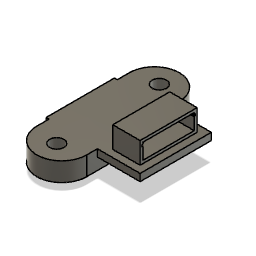
TOF_2D v1 (Autodesk Fusion 360 design; units mm, degrees)
Autodesk Fusion 360 part; units mm, degrees
note: some values were not read from the file. Set by a fixed rule: which sketch regions a step uses.
sketch "草图1" plane through (0, 0, 0) normal (0, 1, 0) x (1, 0, 0)
  line L0 (0, 0) -> (5, 0)
  line L1 (5, 0) -> (5, 9.6)
  line L2 (5, 9.6) -> (0, 9.6)
  line L3 (0, 9.6) -> (0, 0)
  circle A0 centre (2.5, 2.5) radius 2.5
  circle A1 centre (2.5, 7.1) radius 2.5
  dimension "d1" = 5
  dimension "d2" = 9.6
  dimension "d3" = 5
  dimension "d4" = 5
  constraint horizontal L0
  constraint vertical L1
  constraint horizontal L2
  constraint vertical L3
  constraint coincident L0.start L3.end
  constraint tangent L0 A0
  constraint tangent L2 A1
  constraint tangent L1 A1
  measures "d1" distance of L0.start L0.end
  measures "d2" distance of L0.start L2.end
  measures "d3" diameter of A0
  measures "d4" diameter of A1
extrude "拉伸1" add sketch "草图1" along normal blind 1 contours A0 A1 | L3 A0 A1 | L1 A0 A1 | A0 A1 | A0 A1
sketch "草图2" plane through (0, 1, 0) normal (0, 1, 0) x (-1, 0, 0)
  line L0 (1.0001, 5.2) -> (-5.9999, 5.2)
  line L1 (-5.9999, 5.2) -> (-5.9999, -14.8)
  line L2 (-5.9999, -14.8) -> (1.0001, -14.8)
  line L3 (1.0001, -14.8) -> (1.0001, 5.2)
  line L4 (8, -4.8) -> (-8, -4.8)
  line L5 (0, -7.1) -> (0, -2.5)
  line L6 (-2.4999, 15.7777) -> (-2.4999, -15.7777)
  arc A0 (0, -2.5) -> (-5, -2.4998) centre (-2.5, -2.5) ccw
  line L7 (-5.9999, 5.2) -> (1.0001, -14.8)
  line L8 (1.0001, 5.2) -> (-5.9999, -14.8)
  circle A1 centre (-2.4999, -4.8) radius 1.267
  circle A2 centre (-2.4999, -4.8) radius 1.114
  circle A3 centre (-2.4999, 1.7) radius 3.5
  circle A4 centre (-2.4999, -11.3) radius 3.5
  line L9 (1.0001, 5.2) -> (1.0001, 0)
  line L10 (1.0001, 0) -> (1.4001, 0)
  line L11 (1.4001, 0) -> (1.4001, -9.6)
  line L12 (1.4001, -9.6) -> (1.0001, -9.6)
  dimension "d11" = 7
  dimension "d12" = 20
  dimension "d13" = 7
  dimension "d14" = 7
  dimension "d15" = 5.2
  dimension "d19" = 0.4
  dimension "d20" = 9.6
  constraint horizontal L0
  constraint vertical L1
  constraint horizontal L2
  constraint vertical L3
  constraint perpendicular L1 L4
  constraint midpoint L4 L5
  constraint vertical L6
  constraint midpoint L6 A0
  constraint midpoint L8 A1.centre
  constraint coincident L6 A1.centre
  constraint coincident L4 A1.centre
  constraint concentric A1 A2
  constraint tangent L3 A3
  constraint tangent L0 A3
  constraint tangent L3 A4
  constraint tangent L2 A4
  constraint perpendicular L0 L9
  constraint perpendicular L3 L10
  constraint perpendicular L4 L11
  constraint coincident L3 L12.end
  constraint perpendicular L3 L12
  measures "d11" distance of L0.start L0.end
  measures "d12" distance of L0.start L2.end
  measures "d13" diameter of A3
  measures "d14" diameter of A4
  measures "d15" distance of L0.start L9.end
  measures "d19" distance of L9.end L10.end
  measures "d20" distance of L10.end L11.end
extrude "拉伸2" add sketch "草图2" along normal blind 2.65 contours L6 A0 L8 A3 | L6 A0 L7 A3 | A0 L8 A3 | L3 L4 L5 A0 A3 L9 | L6 A0 L8 A3 | L6 A0 L7 A3 | A0 L7 A3 | A0 L8 A3 | L4 L5 A0 L8 A1 A3 | L1 L4 L7 A1 A3 | L6 L8 A1 A3 | L6 L7 A1 A3 | A0 L7 A3 | L3 L4 L7 A1 A4 | L1 L4 L8 A1 A4 | L6 L8 A1 A2 | L6 L7 A1 A2 | L4 L8 A1 A2 | L8 A4 | L4 L7 A1 A2 | L4 L8 A1 A2 | L6 L8 A2 | L6 L7 A2 | L7 A4 | L4 L7 A1 A2 | L4 L8 A2 | L6 L8 A4 | L6 L8 A1 A4 | L4 L7 A2 | L4 L8 A2 | L6 L8 A1 A2 | L6 L7 A2 | L4 L7 A2 | L6 L8 A2 | L6 L7 A1 A4 | L6 L7 A4 | L6 L7 A1 A2
sketch "草图3" plane through (0, 3.65, 0) normal (0, 1, 0) x (-1, 0, 0)
  arc A0 (1.0001, 1.7) -> (-5.9999, 1.7) centre (-2.4999, 1.7) ccw
  line L0 (-5.9999, 1.7) -> (-5.9999, -11.3)
  arc A1 (-5.9999, -11.3) -> (1.0001, -11.3) centre (-2.4999, -11.3) ccw
  line L1 (1.0001, -11.3) -> (1.0001, 1.7)
  line L2 (3.0001, -4.8) -> (-14.9999, -4.8)
  line L3 (-5.9999, 2.4) -> (-5.9999, -12)
  line L4 (-2.4999, 10.5811) -> (-2.4999, -40.1811)
  line L5 (-5.9999, 2.4) -> (-2.4999, 2.4)
  line L6 (-5.9999, -12) -> (-2.4999, -12)
  circle A2 centre (-2.4999, 2.4) radius 1
  circle A3 centre (-2.4999, -12) radius 1
  dimension "d24" = 14.4
  dimension "d25" = 2
  dimension "d26" = 2
  constraint perpendicular L0 L2
  constraint midpoint L0 L2
  constraint vertical L3
  constraint midpoint L2 L3
  constraint vertical L4
  constraint midpoint A1 L4
  constraint coincident L4 L5.end
  constraint perpendicular L4 L5
  constraint coincident L4 L6.end
  constraint perpendicular L4 L6
  constraint coincident L5.end A2.centre
  constraint coincident L6.end A3.centre
  measures "d24" distance of L3.start L3.end
  measures "d25" diameter of A2
  measures "d26" diameter of A3
extrude "拉伸3" cut sketch "草图3" against normal blind 2.65 contours L4 A2 | L4 L5 A2 | L4 L5 A2 | L4 A3 | L4 L6 A3 | L4 L6 A3
sketch "草图5" plane through (0, 3.65, 0) normal (0, 1, 0) x (-1, 0, 0)
  circle A0 centre (-2.4999, 2.4) radius 1
  circle A1 centre (-2.4999, -12) radius 1
  arc A2 (1.0001, 1.7) -> (-5.9999, 1.7) centre (-2.4999, 1.7) ccw
  line L0 (-5.9999, 1.7) -> (-5.9999, -11.3)
  arc A3 (-5.9999, -11.3) -> (1.0001, -11.3) centre (-2.4999, -11.3) ccw
  line L1 (1.0001, -11.3) -> (1.0001, 1.7)
  line L2 (2.5, 5.2) -> (-8.5, 5.2)
  line L3 (1.0001, 1.7) -> (1.0001, 5.2)
  line L4 (-5.9999, 1.7) -> (-5.9999, 5.2)
  line L5 (1.0001, 5.2) -> (1.0001, 0)
  line L6 (-5.9999, 5.2) -> (-5.9999, 0.2)
  line L7 (1.0001, 0) -> (1.4001, 0)
  line L8 (1.4001, 0) -> (1.4001, -9.6)
  line L9 (1.4001, -9.6) -> (1.0001, -9.6)
  line L10 (1.0001, -9.6) -> (1.0001, 0)
  line L11 (-5.9999, 0.2) -> (-11.9999, 0.2)
  line L12 (-11.9999, 0.2) -> (-11.9999, -9.8)
  line L13 (-11.9999, -9.8) -> (-5.9999, -9.8)
  line L14 (-5.9999, -9.8) -> (-5.9999, 0.2)
  dimension "d37" = 5.2
  dimension "d38" = 5
  dimension "d39" = 0.4
  dimension "d40" = 9.6
  dimension "d41" = 6
  dimension "d42" = 10
  constraint horizontal L2
  constraint tangent A2 L2
  constraint coincident A2.start L1.end
  constraint coincident L2 L3.end
  constraint tangent A2 L3
  constraint coincident A2.end L0.start
  constraint coincident L2 L4.end
  constraint tangent A2 L4
  constraint parallel L1 L5
  constraint perpendicular L2 L6
  constraint horizontal L7
  constraint vertical L8
  constraint horizontal L9
  constraint vertical L10
  constraint horizontal L11
  constraint vertical L12
  constraint horizontal L13
  constraint vertical L14
  measures "d37" distance of L3.end L5.end
  measures "d38" distance of L4.end L6.end
  measures "d39" distance of L5.end L7.end
  measures "d40" distance of L5.end L9.end
  measures "d41" distance of L6.end L11.end
  measures "d42" distance of L6.end L13.end
extrude "拉伸4" add sketch "草图5" against normal blind 1 contours L1 L7 L8 L9 L10 | L0 L11 L12 L13 L14
sketch "草图6" plane through (0, 3.65, 0) normal (0, 1, 0) x (-1, 0, 0)
  circle A0 centre (-2.4999, 2.4) radius 1
  circle A1 centre (-2.4999, -12) radius 1
  arc A2 (1.0001, 1.7) -> (-5.9999, 1.7) centre (-2.4999, 1.7) ccw
  line L0 (-5.9999, 1.7) -> (-5.9999, 0.2)
  line L1 (-5.9999, 0.2) -> (-11.9999, 0.2)
  line L2 (-11.9999, 0.2) -> (-11.9999, -9.8)
  line L3 (-11.9999, -9.8) -> (-5.9999, -9.8)
  line L4 (-5.9999, -9.8) -> (-5.9999, -11.3)
  arc A3 (-5.9999, -11.3) -> (1.0001, -11.3) centre (-2.4999, -11.3) ccw
  line L5 (1.0001, -11.3) -> (1.0001, -9.6)
  line L6 (1.0001, -9.6) -> (1.4001, -9.6)
  line L7 (1.4001, -9.6) -> (1.4001, 0)
  line L8 (1.4001, 0) -> (1.0001, 0)
  line L9 (1.0001, 0) -> (1.0001, 1.7)
  line L10 (-11.9999, 0.2) -> (-10.9999, 0.2)
  line L11 (-10.9999, 0.2) -> (-10.9999, -0.8)
  line L12 (-10.9999, -0.8) -> (-11.9999, -0.8)
  line L13 (-11.9999, -0.8) -> (-11.9999, 0.2)
  line L14 (-10.9999, -0.8) -> (-7.1624, -0.8)
  line L15 (-7.1624, -0.8) -> (-7.1624, -8.8)
  line L16 (-7.1624, -8.8) -> (-10.9999, -8.8)
  line L17 (-10.9999, -8.8) -> (-10.9999, -0.8)
  dimension "d46" = 1
  dimension "d47" = 1
  dimension "d48" = 8
  constraint horizontal L10
  constraint vertical L11
  constraint horizontal L12
  constraint vertical L13
  constraint coincident L1.end L2.start
  constraint horizontal L14
  constraint vertical L15
  constraint horizontal L16
  constraint vertical L17
  measures "d46" distance of L1.end L10.end
  measures "d47" distance of L1.end L12.end
  measures "d48" distance of L11.end L16.end
extrude "拉伸5" add sketch "草图6" along normal blind 3 contours L14 L15 L16 L17
sketch "草图7" plane through (10.9999, 0, 0) normal (1, 0, 0) x (0, 0, -1)
  line L0 (0.8, 3.65) -> (8.8, 3.65)
  line L1 (8.8, 3.65) -> (8.8, 6.65)
  line L2 (8.8, 6.65) -> (0.8, 6.65)
  line L3 (0.8, 6.65) -> (0.8, 3.65)
  line L4 (0.8, 6.65) -> (1.2, 6.65)
  line L5 (1.2, 6.65) -> (1.2, 6.25)
  line L6 (1.2, 6.25) -> (0.8, 6.25)
  line L7 (0.8, 6.25) -> (0.8, 6.65)
  line L8 (8.8, 3.65) -> (8.4, 3.65)
  line L9 (8.4, 3.65) -> (8.4, 4.05)
  line L10 (8.4, 4.05) -> (8.8, 4.05)
  line L11 (8.8, 4.05) -> (8.8, 3.65)
  line L12 (1.2, 6.25) -> (8.4, 6.25)
  line L13 (8.4, 6.25) -> (8.4, 4.05)
  line L14 (8.4, 4.05) -> (1.2, 4.05)
  line L15 (1.2, 4.05) -> (1.2, 6.25)
  line L16 (1.2, 6.0193) -> (8.4, 6.0193)
  line L17 (1.2, 5.7535) -> (8.4, 5.7535)
  line L18 (1.2, 5.7535) -> (1.05, 5.7535)
  line L19 (1.2, 6.0193) -> (1.05, 6.0193)
  line L20 (1.05, 6.0193) -> (1.05, 5.7535)
  line L21 (4.8, 10.0193) -> (4.8, 2.0193)
  line L22 (8.55, 5.7535) -> (8.4, 5.7535)
  line L23 (8.55, 6.0193) -> (8.4, 6.0193)
  line L24 (8.55, 5.7535) -> (8.55, 6.0193)
  point P0 (8.55, 6.0193)
  point P1 (8.55, 5.7535)
  dimension "d51" = 0.4
  dimension "d52" = 0.4
  dimension "d53" = 0.4
  dimension "d54" = 0.4
  dimension "d55" = 0.15
  dimension "d56" = 0.15
  constraint horizontal L4
  constraint vertical L5
  constraint horizontal L6
  constraint vertical L7
  constraint coincident L2.end L3.start
  constraint horizontal L8
  constraint vertical L9
  constraint horizontal L10
  constraint vertical L11
  constraint coincident L0.end L1.start
  constraint horizontal L12
  constraint vertical L13
  constraint horizontal L14
  constraint vertical L15
  constraint coincident L15 L16.start
  constraint coincident L13 L16.end
  constraint perpendicular L13 L16
  constraint coincident L15 L17.start
  constraint coincident L13 L17.end
  constraint perpendicular L13 L17
  constraint horizontal L18
  constraint horizontal L19
  constraint perpendicular L0 L21
  constraint midpoint L16 L21
  constraint symmetric L18.end L21 P1
  constraint symmetric L19.end L21 P0
  constraint coincident P1 L22.start
  constraint coincident P0 L23.start
  constraint perpendicular L23 L24
  measures "d51" distance of L2.end L4.end
  measures "d52" distance of L2.end L6.end
  measures "d53" distance of L0.end L8.end
  measures "d54" distance of L0.end L10.end
  measures "d55" distance of L17.start L18.end
  measures "d56" distance of L16.start L19.end
extrude "拉伸6" cut sketch "草图7" against normal blind 3.438 contours L13 L14 L17 L21 | L14 L15 L17 L21 | L13 L16 L17 L21 | L13 L22 L23 L24 | L15 L16 L17 L21 | L12 L13 L16 L21 | L12 L15 L16 L21 | L15 L18 L19 L20
